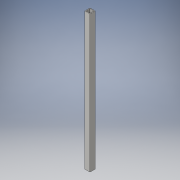
# Autodesk Inventor part: 26 inch 8th inch thick tube
Saved by Autodesk Inventor 2016 (Build 200138000, 138)
## iProperties
Created: 2016-02-05
Part Number: 26 inch 8th inch thick tube
Material: Generic
Document SubType Name: Modeling
Designer: gus
Density: 1 g/cm^3
Appearance: Default
Author: gus
Autodesk Inventor part; units mm, degrees
ref_plane "YZ Plane" through (0, 0, 0) normal (1, 0, 0) x (0, 1, 0)
ref_plane "XZ Plane" through (0, 0, 0) normal (0, 1, 0) x (-1, 0, 0)
ref_plane "XY Plane" through (0, 0, 0) normal (0, 0, 1) x (1, 0, 0)
sketch "Sketch1" plane through (0, 0, 0) normal (0, 1, 0) x (-1, 0, 0)
  line L0 (-1.9439, 0) -> (23.4561, 0)
  line L1 (23.4561, 0) -> (23.4561, 25.4)
  line L2 (23.4561, 25.4) -> (-1.9439, 25.4)
  line L3 (-1.9439, 25.4) -> (-1.9439, 0)
  line L4 (20.2811, 22.225) -> (1.2311, 22.225)
  line L5 (1.2311, 22.225) -> (1.2311, 3.175)
  line L6 (1.2311, 3.175) -> (20.2811, 3.175)
  line L7 (20.2811, 3.175) -> (20.2811, 22.225)
  point P0 (0, 0)
  dimension "d0" = 25.4
  dimension "d1" = 25.4
  dimension "d2" = 3.175
  dimension "d4" = 3.175
  dimension "d5" = 3.175
  dimension "d6" = 3.175
  constraints: 16 end point, 4 parallel, 2 horizontal, 2 perpendicular
  measures "d0" distance of L0.start L0.end
  measures "d1" distance of L2.end L0.start
  measures "d2" distance between parallel lines of L3 L5
  measures "d4" distance between parallel lines of L2 L4
  measures "d5" distance between parallel lines of L0 L6
  measures "d6" distance between parallel lines of L1 L7
extrude "Extrusion1" add sketch "Sketch1" along normal blind 660.4
body "Solid1"
